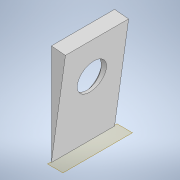
# Autodesk Inventor part: pipeCover02
Saved by Autodesk Inventor 2021.1 (Build 251245000, 245)
## iProperties
Created: 2020-07-06
Part Number: pipeCover02
Material: Generic
Document SubType Name: Modeling
Designer: robst
Density: 1 g/cm^3
Appearance: Default
Author: robst
Autodesk Inventor part; units mm, degrees
ref_plane "YZ Plane" through (0, 0, 0) normal (1, 0, 0) x (0, 1, 0)
ref_plane "XY Plane" through (0, 0, 0) normal (0, 0, 1) x (1, 0, 0)
sketch "Sketch1" plane through (0, 0, 0) normal (0, 0, 1) x (1, 0, 0)
  line L0 (0, 0) -> (14.2789, 101.6)
  line L1 (14.2789, 101.6) -> (0, 101.6)
  line L2 (0, 101.6) -> (0, 0)
  dimension "height" = 101.6
  dimension "d1" = 8
  dimension "d2" = 14.279
  constraints: 6 end point, 1 horizontal, 1 vertical
  measures "height" distance from line of L0.start L1
  measures "d1" angle of L0 L2
  measures "d2" distance of L0.end L1.end
extrude "MainStructure" add sketch "Sketch1" along normal mid plane 63.5
sketch "Sketch2" plane through (0, 0, 31.75) normal (-1, 0, 0) x (0, 0, 1)
  circle A0 centre (-31.75, 63.5) radius 14.605
  line L0 (-63.5, 101.6) -> (0, 101.6) projected
  line L1 (-31.75, 101.6) -> (-31.75, 0) construction
  dimension "hole" = 29.21
  dimension "x" = 38.1
  dimension "d29" = 0
  constraints: 2 end point, 1 centre point, 1 midpoint, 1 vertical
  measures "hole" diameter of A0
  measures "x" distance from line of A0.centre L0
  measures "d29" distance from line of A0.centre L1
extrude "PipeHole" cut sketch "Sketch2" against normal through all
sketch "Sketch6" plane through (0, 0, 0) normal (0, 0, 1) x (1, 0, 0)
  line L0 (0, 101.6) -> (14.2789, 101.6) projected
  line L1 (0, 0) -> (0, 101.6) projected
  line L2 (14.2789, 101.6) -> (0, 0) projected
  line L3 (0, 101.6) -> (14.1055, 100.3659)
  line L4 (14.1055, 100.3659) -> (14.2789, 101.6)
  line L5 (14.2789, 101.6) -> (0, 101.6)
  dimension "mainAngle" = 5
  constraints: 6 end point, 1 collinear, 1 point on line
  measures "mainAngle" angle of L3 L0
extrude "AngleForTopRelief" cut sketch "Sketch6" along normal through all both and the other way through all contours L0 L2 L3
sketch "Sketch7" plane through (0, 0, -31.75) normal (-1, 0, 0) x (0, 0, 1)
  line L0 (0, 0) -> (0, 101.6) construction
  line L1 (0, 31.75) -> (63.5, 31.75) construction
  line L2 (63.5, 0) -> (63.5, 100.3659) construction
  line L3 (0, 0) -> (63.5, 0) projected
  spline S0 degree 2 poles (20.8871, 29.3006) (20.8871, 28.3537) (20.1667, 26.9026) (19.5697, 26.4292) knots 0 0 0 1 2 2 2
  spline S1 degree 2 poles (19.5697, 26.4292) (18.8493, 25.8734) (17.2129, 25.4) (15.9162, 25.4) knots 0 0 0 1 2 2 2
  line L4 (15.9162, 25.4) -> (12.2729, 25.4)
  line L5 (12.2729, 25.4) -> (12.2729, 38.1)
  line L6 (12.2729, 38.1) -> (15.6383, 38.1)
  spline S2 degree 2 poles (15.6383, 38.1) (16.9968, 38.1) (18.3553, 37.925) (18.9728, 37.5854) knots 0 0 0 1 2 2 2
  spline S3 degree 2 poles (18.9728, 37.5854) (19.6624, 37.2252) (20.2902, 36.0417) (20.2902, 35.2389) knots 0 0 0 1 2 2 2
  spline S4 degree 2 poles (20.2902, 35.2389) (20.2902, 34.3435) (19.3433, 32.9233) (18.5097, 32.5219) knots 0 0 0 1 2 2 2
  line L7 (18.5097, 32.5219) -> (18.5097, 32.4601)
  spline S5 degree 2 poles (18.5097, 32.4601) (19.6418, 32.1514) (20.8871, 30.515) (20.8871, 29.3006) knots 0 0 0 1 2 2 2
  spline S6 degree 2 poles (19.1272, 29.2285) (19.1272, 29.9489) (18.7155, 30.8752) (18.098, 31.2045) knots 0 0 0 1 2 2 2
  spline S7 degree 2 poles (18.098, 31.2045) (17.6966, 31.4104) (16.7498, 31.5339) (15.875, 31.5339) knots 0 0 0 1 2 2 2
  line L8 (15.875, 31.5339) -> (13.9607, 31.5339)
  line L9 (13.9607, 31.5339) -> (13.9607, 26.8408)
  line L10 (13.9607, 26.8408) -> (15.3295, 26.8408)
  spline S8 degree 2 poles (15.3295, 26.8408) (16.441, 26.8408) (17.7172, 27.0467) (18.2112, 27.376) knots 0 0 0 1 2 2 2
  spline S9 degree 2 poles (18.2112, 27.376) (18.6846, 27.7156) (19.1272, 28.5596) (19.1272, 29.2285) knots 0 0 0 1 2 2 2
  spline S10 degree 2 poles (18.5303, 35.0022) (18.5303, 35.455) (18.2215, 36.1343) (17.8819, 36.3298) knots 0 0 0 1 2 2 2
  spline S11 degree 2 poles (17.8819, 36.3298) (17.4702, 36.5562) (16.4719, 36.6592) (15.5765, 36.6592) knots 0 0 0 1 2 2 2
  line L11 (15.5765, 36.6592) -> (13.9607, 36.6592)
  line L12 (13.9607, 36.6592) -> (13.9607, 32.9438)
  line L13 (13.9607, 32.9438) -> (15.875, 32.9438)
  spline S12 degree 2 poles (15.875, 32.9438) (16.6675, 32.9438) (17.4188, 33.1085) (17.8201, 33.3658) knots 0 0 0 1 2 2 2
  spline S13 degree 2 poles (17.8201, 33.3658) (18.2112, 33.6128) (18.5303, 34.4053) (18.5303, 35.0022) knots 0 0 0 1 2 2 2
  line L14 (21.1958, 25.4) -> (25.4772, 38.1)
  line L15 (25.4772, 38.1) -> (27.5561, 38.1)
  line L16 (27.5561, 38.1) -> (31.8375, 25.4)
  line L17 (31.8375, 25.4) -> (30.057, 25.4)
  line L18 (30.057, 25.4) -> (28.9043, 28.9506)
  line L19 (28.9043, 28.9506) -> (24.0569, 28.9506)
  line L20 (24.0569, 28.9506) -> (22.9043, 25.4)
  line L21 (22.9043, 25.4) -> (21.1958, 25.4)
  line L22 (28.4412, 30.3915) -> (26.4755, 36.371)
  line L23 (26.4755, 36.371) -> (24.5201, 30.3915)
  line L24 (24.5201, 30.3915) -> (28.4412, 30.3915)
  spline S14 degree 2 poles (38.1669, 25.1736) (36.9319, 25.1736) (34.8427, 26.0072) (34.0811, 26.8408) knots 0 0 0 1 2 2 2
  spline S15 degree 2 poles (34.0811, 26.8408) (33.3195, 27.6642) (32.4859, 30.1342) (32.4859, 31.7397) knots 0 0 0 1 2 2 2
  spline S16 degree 2 poles (32.4859, 31.7397) (32.4859, 33.3349) (33.2989, 35.702) (34.0708, 36.5768) knots 0 0 0 1 2 2 2
  spline S17 degree 2 poles (34.0708, 36.5768) (34.8324, 37.431) (36.9113, 38.3264) (38.1978, 38.3264) knots 0 0 0 1 2 2 2
  spline S18 degree 2 poles (38.1978, 38.3264) (38.8359, 38.3264) (39.9577, 38.1412) (40.4311, 37.9971) knots 0 0 0 1 2 2 2
  spline S19 degree 2 poles (40.4311, 37.9971) (40.8427, 37.8633) (41.697, 37.4825) (42.1189, 37.2561) knots 0 0 0 1 2 2 2
  line L25 (42.1189, 37.2561) -> (42.1189, 35.2183)
  line L26 (42.1189, 35.2183) -> (41.9851, 35.2183)
  spline S20 degree 2 poles (41.9851, 35.2183) (41.7587, 35.4241) (41.0589, 36.0005) (40.5546, 36.2784) knots 0 0 0 1 2 2 2
  spline S21 degree 2 poles (40.5546, 36.2784) (40.0709, 36.5459) (38.9285, 36.8856) (38.1875, 36.8856) knots 0 0 0 1 2 2 2
  spline S22 degree 2 poles (38.1875, 36.8856) (37.3744, 36.8856) (35.9233, 36.2166) (35.3778, 35.5785) knots 0 0 0 1 2 2 2
  spline S23 degree 2 poles (35.3778, 35.5785) (34.8427, 34.9301) (34.2457, 32.9644) (34.2457, 31.7397) knots 0 0 0 1 2 2 2
  spline S24 degree 2 poles (34.2457, 31.7397) (34.2457, 30.4327) (34.8735, 28.5493) (35.419, 27.9009) knots 0 0 0 1 2 2 2
  spline S25 degree 2 poles (35.419, 27.9009) (35.9542, 27.2731) (37.3847, 26.635) (38.1875, 26.635) knots 0 0 0 1 2 2 2
  spline S26 degree 2 poles (38.1875, 26.635) (38.9182, 26.635) (40.1635, 26.9952) (40.6472, 27.2628) knots 0 0 0 1 2 2 2
  spline S27 degree 2 poles (40.6472, 27.2628) (41.1103, 27.5304) (41.7999, 28.0861) (41.9954, 28.2817) knots 0 0 0 1 2 2 2
  line L27 (41.9954, 28.2817) -> (42.1189, 28.2817)
  line L28 (42.1189, 28.2817) -> (42.1189, 26.2645)
  spline S28 degree 2 poles (42.1189, 26.2645) (41.697, 26.069) (40.956, 25.7088) (40.4311, 25.5441) knots 0 0 0 1 2 2 2
  spline S29 degree 2 poles (40.4311, 25.5441) (39.8753, 25.3588) (38.9285, 25.1736) (38.1669, 25.1736) knots 0 0 0 1 2 2 2
  line L29 (52.9561, 25.4) -> (50.764, 25.4)
  line L30 (50.764, 25.4) -> (46.1224, 31.3075)
  line L31 (46.1224, 31.3075) -> (45.3814, 30.4738)
  line L32 (45.3814, 30.4738) -> (45.3814, 25.4)
  line L33 (45.3814, 25.4) -> (43.6936, 25.4)
  line L34 (43.6936, 25.4) -> (43.6936, 38.1)
  line L35 (43.6936, 38.1) -> (45.3814, 38.1)
  line L36 (45.3814, 38.1) -> (45.3814, 32.2646)
  line L37 (45.3814, 32.2646) -> (50.589, 38.1)
  line L38 (50.589, 38.1) -> (52.6474, 38.1)
  line L39 (52.6474, 38.1) -> (47.3883, 32.4293)
  line L40 (47.3883, 32.4293) -> (52.9561, 25.4)
  point P0 (31.75, 0)
  dimension "lineForText" = 31.75
  constraints: 2 end point, 2 horizontal, 2 point on line
  measures "lineForText" distance between parallel lines of L3 L1
extrude "TextForBack" cut sketch "Sketch7" against normal blind 1.016
sketch "Sketch8" plane through (0, 0, -31.75) normal (-1, 0, 0) x (0, 0, 1)
  circle A0 centre (31.75, 63.5) radius 14.605 projected
  circle A1 centre (31.75, 63.5) radius 19.05
  point P0 (31.75, 0)
  dimension "reliefHoleDiameter" = 38.1
  constraints: 1 centre point, 1 coincident
  measures "reliefHoleDiameter" diameter of A1
extrude "ReliefForHole" cut sketch "Sketch8" against normal blind 3.81 contours A0 | A1
sketch "Sketch9" plane through (0, 0, -31.75) normal (-1, 0, 0) x (0, 0, 1)
  line L0 (0, 100.3659) -> (0, 0) projected
  line L1 (0, 92.075) -> (63.5, 92.075) construction
  line L2 (63.5, 0) -> (63.5, 100.3659) projected
  line L3 (0, 101.6) -> (63.5, 101.6) construction
  spline S0 degree 2 poles (17.4664, 90.2379) (17.4664, 89.5278) (16.926, 88.4394) (16.4784, 88.0844) knots 0 0 0 1 2 2 2
  spline S1 degree 2 poles (16.4784, 88.0844) (15.938, 87.6676) (14.7107, 87.3125) (13.7382, 87.3125) knots 0 0 0 1 2 2 2
  line L4 (13.7382, 87.3125) -> (11.0057, 87.3125)
  line L5 (11.0057, 87.3125) -> (11.0057, 96.8375)
  line L6 (11.0057, 96.8375) -> (13.5298, 96.8375)
  spline S2 degree 2 poles (13.5298, 96.8375) (14.5487, 96.8375) (15.5675, 96.7063) (16.0307, 96.4516) knots 0 0 0 1 2 2 2
  spline S3 degree 2 poles (16.0307, 96.4516) (16.5478, 96.1814) (17.0187, 95.2937) (17.0187, 94.6917) knots 0 0 0 1 2 2 2
  spline S4 degree 2 poles (17.0187, 94.6917) (17.0187, 94.0201) (16.3085, 92.9549) (15.6833, 92.6539) knots 0 0 0 1 2 2 2
  line L7 (15.6833, 92.6539) -> (15.6833, 92.6076)
  spline S5 degree 2 poles (15.6833, 92.6076) (16.5324, 92.376) (17.4664, 91.1487) (17.4664, 90.2379) knots 0 0 0 1 2 2 2
  spline S6 degree 2 poles (16.1464, 90.1839) (16.1464, 90.7242) (15.8377, 91.4189) (15.3746, 91.6659) knots 0 0 0 1 2 2 2
  spline S7 degree 2 poles (15.3746, 91.6659) (15.0735, 91.8203) (14.3634, 91.9129) (13.7073, 91.9129) knots 0 0 0 1 2 2 2
  line L8 (13.7073, 91.9129) -> (12.2716, 91.9129)
  line L9 (12.2716, 91.9129) -> (12.2716, 88.3931)
  line L10 (12.2716, 88.3931) -> (13.2982, 88.3931)
  spline S8 degree 2 poles (13.2982, 88.3931) (14.1318, 88.3931) (15.089, 88.5475) (15.4595, 88.7945) knots 0 0 0 1 2 2 2
  spline S9 degree 2 poles (15.4595, 88.7945) (15.8145, 89.0492) (16.1464, 89.6822) (16.1464, 90.1839) knots 0 0 0 1 2 2 2
  spline S10 degree 2 poles (15.6988, 94.5141) (15.6988, 94.8538) (15.4672, 95.3632) (15.2125, 95.5099) knots 0 0 0 1 2 2 2
  spline S11 degree 2 poles (15.2125, 95.5099) (14.9037, 95.6797) (14.155, 95.7569) (13.4835, 95.7569) knots 0 0 0 1 2 2 2
  line L11 (13.4835, 95.7569) -> (12.2716, 95.7569)
  line L12 (12.2716, 95.7569) -> (12.2716, 92.9704)
  line L13 (12.2716, 92.9704) -> (13.7073, 92.9704)
  spline S12 degree 2 poles (13.7073, 92.9704) (14.3017, 92.9704) (14.8651, 93.0939) (15.1662, 93.2869) knots 0 0 0 1 2 2 2
  spline S13 degree 2 poles (15.1662, 93.2869) (15.4595, 93.4721) (15.6988, 94.0665) (15.6988, 94.5141) knots 0 0 0 1 2 2 2
  line L14 (21.7889, 87.3125) -> (24.9999, 96.8375)
  line L15 (24.9999, 96.8375) -> (26.5591, 96.8375)
  line L16 (26.5591, 96.8375) -> (29.7701, 87.3125)
  line L17 (29.7701, 87.3125) -> (28.4348, 87.3125)
  line L18 (28.4348, 87.3125) -> (27.5703, 89.9755)
  line L19 (27.5703, 89.9755) -> (23.9347, 89.9755)
  line L20 (23.9347, 89.9755) -> (23.0702, 87.3125)
  line L21 (23.0702, 87.3125) -> (21.7889, 87.3125)
  line L22 (27.2229, 91.0561) -> (25.7486, 95.5407)
  line L23 (25.7486, 95.5407) -> (24.2821, 91.0561)
  line L24 (24.2821, 91.0561) -> (27.2229, 91.0561)
  spline S14 degree 2 poles (38.6082, 87.1427) (37.6819, 87.1427) (36.115, 87.7679) (35.5438, 88.3931) knots 0 0 0 1 2 2 2
  spline S15 degree 2 poles (35.5438, 88.3931) (34.9726, 89.0106) (34.3474, 90.8631) (34.3474, 92.0673) knots 0 0 0 1 2 2 2
  spline S16 degree 2 poles (34.3474, 92.0673) (34.3474, 93.2637) (34.9572, 95.039) (35.5361, 95.6951) knots 0 0 0 1 2 2 2
  spline S17 degree 2 poles (35.5361, 95.6951) (36.1073, 96.3358) (37.6665, 97.0073) (38.6313, 97.0073) knots 0 0 0 1 2 2 2
  spline S18 degree 2 poles (38.6313, 97.0073) (39.1099, 97.0073) (39.9512, 96.8684) (40.3063, 96.7603) knots 0 0 0 1 2 2 2
  spline S19 degree 2 poles (40.3063, 96.7603) (40.615, 96.66) (41.2557, 96.3744) (41.5722, 96.2046) knots 0 0 0 1 2 2 2
  line L25 (41.5722, 96.2046) -> (41.5722, 94.6762)
  line L26 (41.5722, 94.6762) -> (41.4718, 94.6762)
  spline S20 degree 2 poles (41.4718, 94.6762) (41.302, 94.8306) (40.7771, 95.2629) (40.3989, 95.4713) knots 0 0 0 1 2 2 2
  spline S21 degree 2 poles (40.3989, 95.4713) (40.0361, 95.672) (39.1793, 95.9267) (38.6236, 95.9267) knots 0 0 0 1 2 2 2
  spline S22 degree 2 poles (38.6236, 95.9267) (38.0138, 95.9267) (36.9255, 95.425) (36.5164, 94.9464) knots 0 0 0 1 2 2 2
  spline S23 degree 2 poles (36.5164, 94.9464) (36.115, 94.4601) (35.6673, 92.9858) (35.6673, 92.0673) knots 0 0 0 1 2 2 2
  spline S24 degree 2 poles (35.6673, 92.0673) (35.6673, 91.087) (36.1381, 89.6745) (36.5472, 89.1882) knots 0 0 0 1 2 2 2
  spline S25 degree 2 poles (36.5472, 89.1882) (36.9486, 88.7173) (38.0215, 88.2388) (38.6236, 88.2388) knots 0 0 0 1 2 2 2
  spline S26 degree 2 poles (38.6236, 88.2388) (39.1716, 88.2388) (40.1056, 88.5089) (40.4684, 88.7096) knots 0 0 0 1 2 2 2
  spline S27 degree 2 poles (40.4684, 88.7096) (40.8157, 88.9103) (41.3329, 89.3271) (41.4795, 89.4738) knots 0 0 0 1 2 2 2
  line L27 (41.4795, 89.4738) -> (41.5722, 89.4738)
  line L28 (41.5722, 89.4738) -> (41.5722, 87.9609)
  spline S28 degree 2 poles (41.5722, 87.9609) (41.2557, 87.8142) (40.7, 87.5441) (40.3063, 87.4206) knots 0 0 0 1 2 2 2
  spline S29 degree 2 poles (40.3063, 87.4206) (39.8895, 87.2816) (39.1793, 87.1427) (38.6082, 87.1427) knots 0 0 0 1 2 2 2
  line L29 (53.791, 87.3125) -> (52.1469, 87.3125)
  line L30 (52.1469, 87.3125) -> (48.6658, 91.7431)
  line L31 (48.6658, 91.7431) -> (48.11, 91.1179)
  line L32 (48.11, 91.1179) -> (48.11, 87.3125)
  line L33 (48.11, 87.3125) -> (46.8441, 87.3125)
  line L34 (46.8441, 87.3125) -> (46.8441, 96.8375)
  line L35 (46.8441, 96.8375) -> (48.11, 96.8375)
  line L36 (48.11, 96.8375) -> (48.11, 92.4609)
  line L37 (48.11, 92.4609) -> (52.0157, 96.8375)
  line L38 (52.0157, 96.8375) -> (53.5595, 96.8375)
  line L39 (53.5595, 96.8375) -> (49.6152, 92.5844)
  line L40 (49.6152, 92.5844) -> (53.791, 87.3125)
  point P0 (31.75, 0)
  dimension "d35" = 9.525
  constraints: 2 end point, 2 horizontal, 2 point on line
  measures "d35" distance between parallel lines of L1 L3
extrude "TextForSmallText" cut sketch "Sketch9" against normal blind 1.016
sketch "Sketch10" plane through (14.1055, 100.3659, 31.75) normal (0.0871557, 0.9961947, 0) x (0.9961947, -0.0871557, 0)
  line L0 (-14.1594, 63.5) -> (-14.1594, 0) projected
  line L1 (0, 0) -> (-14.1594, 0) projected
  line L2 (0, 63.5) -> (0, 0) projected
  line L3 (-14.1594, 0) -> (0, 14.1594)
  line L4 (-14.1594, 0) -> (5.865, 0) construction
  line L5 (0, 14.1594) -> (0, 0)
  line L6 (0, 0) -> (-14.1594, 0)
  line L7 (-14.1594, 63.5) -> (0, 63.5) projected
  line L8 (-14.1594, 63.5) -> (0, 49.3406)
  line L9 (-14.1594, 63.5) -> (5.865, 63.5) construction
  line L10 (0, 49.3406) -> (0, 63.5)
  line L11 (0, 63.5) -> (-14.1594, 63.5)
  point P0 (-5.3044, 31.75)
  dimension "d38" = 45
  dimension "d39" = 45
  constraints: 16 end point, 2 collinear, 2 equal length, 2 horizontal, 2 point on line
  measures "d38" angle of L4 L3
  measures "d39" angle of L8 L9
equation "\"depthForText\" = textDepth"
equation "\"d36\" = textDepth"
equation "\"textDepth\" = 1.016"
body "Solid1"
